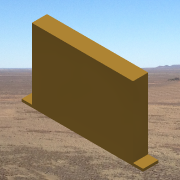
# Autodesk Inventor part: pam
Saved by Autodesk Inventor 2014 SP1 (Build 180222100, 222)
## iProperties
Created: 2014-05-23
Part Number: pam
Material: Brass, Soft Yellow
Document SubType Name: Modeling
Designer: Dave
Density: 8.47 g/cm^3
Appearance: Brass - Satin
Mass: 15198.4 g
Surface Area: 1314.51 cm^2
Volume: 1794.38 cm^3
Author: Dave
Autodesk Inventor part; units mm, degrees
ref_plane "YZ Plane" through (0, 0, 0) normal (1, 0, 0) x (0, 1, 0)
ref_plane "XZ Plane" through (0, 0, 0) normal (0, 1, 0) x (-1, 0, 0)
ref_plane "XY Plane" through (0, 0, 0) normal (0, 0, 1) x (1, 0, 0)
sketch "Sketch1" plane through (0, 0, 0) normal (0, 0, 1) x (1, 0, 0)
  line L0 (0, 0) -> (304.8, 0)
  line L1 (304.8, 0) -> (304.8, 6.35)
  line L2 (304.8, 6.35) -> (279.4, 6.35)
  line L3 (279.4, 6.35) -> (279.4, 184.15)
  line L4 (152.4, 0) -> (152.4, 43.3584) construction
  line L5 (0, 0) -> (0, 6.35)
  line L6 (0, 6.35) -> (25.4, 6.35)
  line L7 (25.4, 6.35) -> (25.4, 184.15)
  line L8 (25.4, 184.15) -> (279.4, 184.15)
  dimension "d0" = 304.8
  dimension "d1" = 6.35
  dimension "d2" = 25.4
  dimension "d3" = 177.8
  constraints: 18 end point, 3 perpendicular, 3 symmetric about line, 2 parallel, 1 horizontal, 1 midpoint
  measures "d0" distance of L0.start L0.end
  measures "d1" distance of L0.end L1.end
  measures "d2" distance of L1.end L2.end
  measures "d3" distance of L2.end L3.end
extrude "Extrusion1" add sketch "Sketch1" along normal blind 38.1
body "Solid1"
